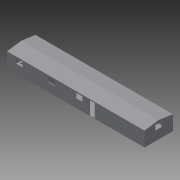
# Autodesk Inventor part: Manufactured_Home_Drawing
Saved by Autodesk Inventor 2013 SP2 (Build 170200200, 200)
## iProperties
Created: 2014-01-20
Part Number: Manufactured_Home_Drawing
Material: Generic
Document SubType Name: Modeling
Designer: mcgratta
Density: 1 g/cm^3
Author: mcgratta
Autodesk Inventor part; units mm, degrees
ref_plane "YZ Plane" through (0, 0, 0) normal (1, 0, 0) x (0, 1, 0)
ref_plane "XZ Plane" through (0, 0, 0) normal (0, 1, 0) x (-1, 0, 0)
ref_plane "XY Plane" through (0, 0, 0) normal (0, 0, 1) x (1, 0, 0)
sketch "Sketch1" plane through (0, 0, 0) normal (0, 1, 0) x (-1, 0, 0)
  line L0 (0, 0) -> (-20120, 0)
  line L1 (-20120, 0) -> (-20120, -4160)
  line L2 (-20120, -4160) -> (0, -4160)
  line L3 (0, -4160) -> (0, 0)
  dimension "d0" = 20120
  dimension "d2" = 4160
  constraints: 8 end point, 2 parallel, 1 horizontal, 1 perpendicular
  measures "d0" distance between parallel lines of L1 L3
  measures "d2" distance between parallel lines of L0 L2
extrude "Extrusion1" add sketch "Sketch1" along normal blind 10
sketch "Sketch5" plane through (0, 0, -4160) normal (-1, 0, 0) x (0, 0, 1)
  line L0 (0, 10) -> (4160, 10)
  line L1 (4160, 10) -> (4160, 2110)
  line L2 (4160, 2110) -> (0, 2110)
  line L3 (0, 2110) -> (0, 10)
  line L4 (0, 2110) -> (2080, 2410)
  line L5 (2080, 2410) -> (4160, 2110)
  line L6 (4160, 2141.0377) -> (2080, 2441.0377)
  line L7 (2080, 2441.0377) -> (0, 2141.0377)
  line L8 (4160, 2110) -> (4160, 2141.0377)
  line L9 (0, 2141.0377) -> (0, 2110)
  dimension "d11" = 2100
  dimension "d12" = 4160
  dimension "d13" = 2080
  dimension "d14" = 2080
  dimension "d15" = 0
  dimension "d16" = 300
  dimension "d17" = 0
  constraints: 20 end point, 5 parallel, 1 horizontal, 1 perpendicular
  measures "d11" distance of L2.end L0.start
  measures "d12" distance between parallel lines of L1 L3
  measures "d13" horizontal distance of L2.end L4.end
  measures "d14" horizontal distance of L6.end L7.end
  measures "d15" horizontal distance of L1.end L6.start
  measures "d16" distance from line of L2 L4.end
  measures "d17" horizontal distance of L2.end L7.end
extrude "Extrusion2" add sketch "Sketch5" against normal blind 20120 contours L9 L7 L6 L8 L5 L4
sketch "Sketch6" plane through (0, 10, 0) normal (0, 1, 0) x (1, 0, 0)
  line L0 (0, 0) -> (20120, 0) projected
  line L1 (20120, 0) -> (20120, 4160) projected
  line L2 (20120, 4160) -> (0, 4160) projected
  line L3 (0, 0) -> (20120, 0)
  line L4 (20120, 0) -> (20120, 4160)
  line L5 (20120, 4160) -> (0, 4160)
  line L6 (0, 4160) -> (0, 0)
  line L7 (100, 100) -> (20020, 100)
  line L8 (20020, 100) -> (20020, 4060)
  line L9 (20020, 4060) -> (100, 4060)
  line L10 (100, 4060) -> (100, 100)
  line L11 (3580, 100) -> (3480, 100)
  line L12 (3480, 100) -> (3480, 2330)
  line L13 (3480, 2330) -> (3580, 2330)
  line L14 (3580, 2330) -> (3580, 100)
  line L15 (5740, 100) -> (5640, 100)
  line L16 (5640, 100) -> (5640, 2330)
  line L17 (5640, 2330) -> (5740, 2330)
  line L18 (5740, 2330) -> (5740, 100)
  line L19 (3580, 2330) -> (3984.3421, 2330)
  line L20 (3984.3421, 2330) -> (3984.3421, 2230)
  line L21 (3984.3421, 2230) -> (3580, 2230)
  line L22 (3580, 2230) -> (3580, 2330)
  line L23 (5640, 2330) -> (4889.9542, 2330)
  line L24 (4889.9542, 2330) -> (4889.9542, 2230)
  line L25 (4889.9542, 2230) -> (5640, 2230)
  line L26 (5640, 2230) -> (5640, 2330)
  line L27 (3480, 4060) -> (3580, 4060)
  line L28 (3580, 4060) -> (3580, 3450)
  line L29 (3580, 3450) -> (3480, 3450)
  line L30 (3480, 3450) -> (3480, 4060)
  line L31 (3480, 3450) -> (2389.9015, 3450)
  line L32 (2389.9015, 3450) -> (2389.9015, 3550)
  line L33 (2389.9015, 3550) -> (3480, 3550)
  line L34 (3480, 3550) -> (3480, 3450)
  line L35 (100, 3450) -> (1181.4833, 3450)
  line L36 (1181.4833, 3450) -> (1181.4833, 3550)
  line L37 (1181.4833, 3550) -> (100, 3550)
  line L38 (100, 3550) -> (100, 3450)
  line L39 (17430, 4060) -> (17330, 4060)
  line L40 (17330, 4060) -> (17330, 2290)
  line L41 (17330, 2290) -> (17430, 2290)
  line L42 (17430, 2290) -> (17430, 4060)
  line L43 (17330, 2490) -> (15650, 2490)
  line L44 (15650, 2490) -> (15650, 2590)
  line L45 (15650, 2590) -> (17330, 2590)
  line L46 (17330, 2590) -> (17330, 2490)
  line L47 (15246.2145, 1020) -> (17430, 1020)
  line L48 (17430, 1020) -> (17430, 920)
  line L49 (17430, 920) -> (15246.2145, 920)
  line L50 (15246.2145, 920) -> (15246.2145, 1020)
  line L51 (17430, 1020) -> (17330, 1020)
  line L52 (17330, 1020) -> (17330, 1519.304)
  line L53 (17330, 1519.304) -> (17430, 1519.304)
  line L54 (17430, 1519.304) -> (17430, 1020)
  line L55 (15650, 3017.3001) -> (15550, 3017.3001)
  line L56 (15550, 3017.3001) -> (15550, 1020)
  line L57 (15550, 1020) -> (15650, 1020)
  line L58 (15650, 1020) -> (15650, 3017.3001)
  line L59 (15550, 4060) -> (15650, 4060)
  line L60 (15650, 4060) -> (15650, 3753.7451)
  line L61 (15650, 3753.7451) -> (15550, 3753.7451)
  line L62 (15550, 3753.7451) -> (15550, 4060)
  line L63 (13210, 4060) -> (13110, 4060)
  line L64 (13110, 4060) -> (13110, 920)
  line L65 (13110, 920) -> (13210, 920)
  line L66 (13210, 920) -> (13210, 4060)
  line L67 (13210, 920) -> (14090.8132, 920)
  line L68 (14090.8132, 920) -> (14090.8132, 1020)
  line L69 (14090.8132, 1020) -> (13210, 1020)
  line L70 (13210, 1020) -> (13210, 920)
  dimension "d20" = 100
  dimension "d22" = 100
  dimension "d23" = 100
  dimension "d24" = 100
  dimension "d25" = 3480
  dimension "d26" = 2230
  dimension "d27" = 100
  dimension "d28" = 2160
  dimension "d29" = 100
  dimension "d30" = 100
  dimension "d31" = 100
  dimension "d32" = 100
  dimension "d33" = 2590
  dimension "d34" = 100
  dimension "d35" = 1770
  dimension "d36" = 1470
  dimension "d37" = 100
  dimension "d38" = 1680
  dimension "d39" = 1470
  dimension "d40" = 100
  dimension "d41" = 100
  dimension "d42" = 2440
  dimension "d43" = 0
  dimension "d44" = 0
  dimension "d45" = 100
  dimension "d48" = 3350
  dimension "d49" = 3350
  dimension "d50" = 3380
  dimension "d51" = 100
  constraints: 136 end point, 34 parallel, 17 horizontal, 17 perpendicular, 9 point on line
  measures "d20" distance between parallel lines of L10 L6
  measures "d22" distance between parallel lines of L9 L2
  measures "d23" distance between parallel lines of L0 L7
  measures "d24" distance between parallel lines of L1 L8
  measures "d25" distance between parallel lines of L14 L10
  measures "d26" distance between parallel lines of L11 L13
  measures "d27" distance between parallel lines of L14 L12
  measures "d28" distance between parallel lines of L18 L14
  measures "d29" distance between parallel lines of L18 L16
  measures "d30" distance between parallel lines of L21 L19
  measures "d31" distance between parallel lines of L31 L33
  measures "d32" distance between parallel lines of L37 L35
  measures "d33" distance between parallel lines of L8 L42
  measures "d34" distance between parallel lines of L42 L40
  measures "d35" distance of L41.end L39.start
  measures "d36" distance between parallel lines of L9 L45
  measures "d37" distance between parallel lines of L43 L45
  measures "d38" distance of L45.end L44.end
  measures "d39" distance between parallel lines of L47 L43
  measures "d40" distance between parallel lines of L49 L47
  measures "d41" distance between parallel lines of L58 L56
  measures "d42" distance between parallel lines of L62 L64
  measures "d43" distance between parallel lines of L62 L56
  measures "d44" distance from line of L44.end L58
  measures "d45" distance between parallel lines of L66 L64
  measures "d48" distance between parallel lines of L7 L35
  measures "d49" distance between parallel lines of L7 L31
  measures "d50" distance between parallel lines of L30 L10
  measures "d51" distance between parallel lines of L28 L30
extrude "Extrusion3" add sketch "Sketch6" along normal up to next contours L6 L2 L1 L0 | L12 L13 L14 L7 | L10 L37 L36 L35 | L16 L17 L18 L7 | L14 L19 L20 L21 | L25 L24 L23 L16 | L9 L28 L29 L30 | L30 L31 L32 L33 | L9 L66 L65 L64 | L42 L41 L40 L9 | L69 L68 L67 L66 | L40 L43 L44 L45 | L44 L58 L47 L56 L55 | L47 L48 L49 L50 | L52 L53 L54 L47
sketch "Sketch7" plane through (20120, 0, 0) normal (1, 0, 0) x (0, 0, -1)
  line L0 (0, 0) -> (4160, 0) projected
  line L1 (1580, 1350) -> (2580, 1350)
  line L2 (2580, 1350) -> (2580, 2050)
  line L3 (2580, 2050) -> (1580, 2050)
  line L4 (1580, 2050) -> (1580, 1350)
  line L5 (1580, 1350) -> (2580, 2050) construction
  line L6 (2580, 1350) -> (1580, 2050) construction
  point P0 (2080, 2441.0377)
  point P1 (2080, 1700)
  dimension "d52" = 1000
  dimension "d54" = 0
  dimension "d55" = 1700
  dimension "d56" = 700
  constraints: 12 end point, 2 midpoint, 2 parallel, 1 horizontal, 1 perpendicular
  measures "d52" distance of L1.start L1.end
  measures "d54" horizontal distance of point (2080, 2441.038) point (2080, 1700)
  measures "d55" distance from line of L0 point (2080, 1700)
  measures "d56" distance between parallel lines of L1 L3
extrude "Extrusion4" cut sketch "Sketch7" along normal mid plane 200
sketch "Sketch8" plane through (0, 0, 0) normal (0, 0, 1) x (1, 0, 0)
  line L0 (0, 0) -> (20120, 0) projected
  line L1 (1300, 1250) -> (2300, 1250)
  line L2 (2300, 1250) -> (2300, 1950)
  line L3 (2300, 1950) -> (1300, 1950)
  line L4 (1300, 1950) -> (1300, 1250)
  line L5 (1300, 1250) -> (2300, 1950) construction
  line L6 (2300, 1250) -> (1300, 1950) construction
  line L7 (100, 10) -> (100, 2124.4231) projected
  line L8 (6000, 1250) -> (7000, 1250)
  line L9 (7000, 1250) -> (7000, 1950)
  line L10 (7000, 1950) -> (6000, 1950)
  line L11 (6000, 1950) -> (6000, 1250)
  line L12 (6000, 1250) -> (7000, 1950) construction
  line L13 (7000, 1250) -> (6000, 1950) construction
  line L14 (10035.7615, 1250) -> (11035.7615, 1250)
  line L15 (11035.7615, 1250) -> (11035.7615, 1950)
  line L16 (11035.7615, 1950) -> (10035.7615, 1950)
  line L17 (10035.7615, 1950) -> (10035.7615, 1250)
  line L18 (10035.7615, 1250) -> (11035.7615, 1950) construction
  line L19 (11035.7615, 1250) -> (10035.7615, 1950) construction
  line L20 (12020, 0) -> (12820, 0)
  line L21 (12820, 0) -> (12820, 2000)
  line L22 (12820, 2000) -> (12020, 2000)
  line L23 (12020, 2000) -> (12020, 0)
  line L24 (20020, 10) -> (20020, 2124.4231) projected
  point P0 (1800, 1600)
  point P1 (6500, 1600)
  point P2 (10535.7615, 1600)
  dimension "d59" = 1700
  dimension "d60" = 1600
  dimension "d61" = 1000
  dimension "d62" = 700
  dimension "d63" = 1000
  dimension "d64" = 700
  dimension "d65" = 1000
  dimension "d66" = 700
  dimension "d67" = 1600
  dimension "d68" = 6400
  dimension "d69" = 2000
  dimension "d70" = 800
  dimension "d71" = 7200
  constraints: 44 end point, 8 parallel, 6 midpoint, 4 horizontal, 4 perpendicular, 1 point on line
  measures "d59" distance from line of L7 point (1800, 1600)
  measures "d60" distance from line of L0 point (1800, 1600)
  measures "d61" distance of L1.start L1.end
  measures "d62" distance of L3.end L1.start
  measures "d63" distance of L8.start L8.end
  measures "d64" distance of L10.end L8.start
  measures "d65" distance of L14.start L14.end
  measures "d66" distance of L16.end L14.start
  measures "d67" distance from line of L0 point (6500, 1600)
  measures "d68" distance from line of L7 point (6500, 1600)
  measures "d69" distance between parallel lines of L20 L22
  measures "d70" distance between parallel lines of L21 L23
  measures "d71" distance between parallel lines of L24 L21
extrude "Extrusion5" cut sketch "Sketch8" along normal mid plane 200
sketch "Sketch9" plane through (0, 10, 0) normal (0, 1, 0) x (1, 0, 0)
  line L0 (12820, 0) -> (20120, 0) projected
  line L1 (20120, 0) -> (20120, 4160) projected
  line L2 (20120, 4160) -> (0, 4160) projected
  line L3 (0, 4160) -> (0, 0) projected
  line L4 (0, 0) -> (12020, 0) projected
  line L5 (280, 1530) -> (680, 1930) construction
  line L6 (680, 1530) -> (280, 1930) construction
  line L7 (3760, 2510) -> (4160, 2910) construction
  line L8 (4160, 2510) -> (3760, 2910) construction
  line L9 (12530, 1500) -> (12930, 1900) construction
  line L10 (12930, 1500) -> (12530, 1900) construction
  line L11 (16750, 430) -> (17150, 830) construction
  line L12 (17150, 430) -> (16750, 830) construction
  line L13 (17610, 1500) -> (18010, 1900) construction
  line L14 (18010, 1500) -> (17610, 1900) construction
  circle A0 centre (480, 1730) radius 196.2005
  circle A1 centre (3960, 2710) radius 200
  circle A2 centre (16950, 630) radius 200
  circle A3 centre (17810, 1700) radius 200
  circle A4 centre (12730, 1700) radius 200
  dimension "d74" = 1730
  dimension "d75" = 480
  dimension "d76" = 400
  dimension "d77" = 400
  dimension "d78" = 400
  dimension "d79" = 400
  dimension "d82" = 400
  dimension "d83" = 400
  dimension "d84" = 400
  dimension "d85" = 400
  dimension "d86" = 3960
  dimension "d87" = 2710
  dimension "d88" = 1700
  dimension "d89" = 7390
  dimension "d90" = 3530
  dimension "d91" = 3170
  dimension "d92" = 2310
  dimension "d93" = 1700
  dimension "d96" = 400
  constraints: 20 end point, 10 midpoint, 5 centre point, 5 coincident
  measures "d74" distance from line of L4 point (480, 1730)
  measures "d75" distance from line of point (480, 1730) L3
  measures "d76" distance of L5.start L6.start
  measures "d77" distance of L6.start L5.end
  measures "d78" distance of L7.start L8.start
  measures "d79" distance of L8.start L7.end
  measures "d82" distance of L11.start L12.start
  measures "d83" distance of L12.start L11.end
  measures "d84" distance of L13.start L14.start
  measures "d85" distance of L14.start L13.end
  measures "d86" distance from line of L3 point (3960, 2710)
  measures "d87" distance from line of L4 point (3960, 2710)
  measures "d88" distance from line of L4 point (12730, 1700)
  measures "d89" distance from line of L1 point (12730, 1700)
  measures "d90" distance from line of L2 point (16950, 630)
  measures "d91" distance from line of L1 point (16950, 630)
  measures "d92" distance from line of L1 point (17810, 1700)
  measures "d93" distance from line of L0 point (17810, 1700)
  measures "d96" diameter of A4
extrude "Extrusion6" add sketch "Sketch9" along normal blind 200
body "Solid1"
